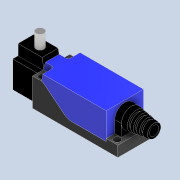
# Autodesk Inventor part: High Voltage Limit Switch
Saved by Autodesk Inventor 2022 (Build 260153000, 153)
## iProperties
Created: 2021-10-24
Part Number: High Voltage Limit Switch
Material: Generic
Document SubType Name: Modeling
Designer: Coy
Density: 1 g/cm^3
Appearance: Anodized - Black
Author: Coy
Autodesk Inventor part; units mm, degrees
ref_plane "YZ Plane" through (0, 0, 0) normal (1, 0, 0) x (0, 1, 0)
sketch "Sketch1" plane through (0, 0, 0) normal (0, 1, 0) x (-1, 0, 0)
  line L0 (0, 0) -> (64, 0)
  line L1 (64, 0) -> (64, 28)
  line L2 (64, 28) -> (0, 28)
  line L3 (0, 28) -> (0, 0)
  dimension "d0" = 64
  dimension "d1" = 28
  constraints: 8 end point, 2 parallel, 1 horizontal, 1 perpendicular
  measures "d0" distance of L1.end L2.end
  measures "d1" distance of L2.end L0.start
extrude "Extrusion1" add sketch "Sketch1" along normal blind 21
sketch "Sketch2" plane through (0, 0, 0) normal (0, 0, -1) x (-1, 0, 0)
  line L0 (0, 0) -> (64, 0) projected
  line L1 (64, 0) -> (64, 21) projected
  line L2 (0, 21) -> (64, 21) projected
  line L3 (0, 0) -> (0, 21) projected
  line L4 (0, 0) -> (0, 21) projected
  line L5 (0, 8) -> (8.75, 8)
  line L6 (0, 0) -> (0, 21) projected
  line L7 (8.75, 6) -> (34.2422, 6)
  line L8 (8.75, 6) -> (8.75, 8)
  line L9 (64, 21) -> (57.2016, 21)
  line L10 (64, 21) -> (0, 21) projected
  line L11 (55.9522, 20.5617) -> (40.4891, 8.1913)
  arc A0 (34.2422, 6) -> (40.4891, 8.1913) centre (34.2422, 16) ccw
  arc A1 (57.2016, 21) -> (55.9522, 20.5617) centre (57.2016, 19) ccw
  point P0 (37.75, 6)
  point P1 (56.5, 21)
  point P2 (57.2016, 21)
  dimension "d4" = 8.75
  dimension "d5" = 8
  dimension "d6" = 29
  dimension "d7" = 2
  dimension "d8" = 7.5
  dimension "d9" = 10
  dimension "d10" = 2
  constraints: 10 end point, 6 point on line, 4 point on circle, 4 tangent, 3 perpendicular, 2 centre point, 1 horizontal
  measures "d4" distance of L5.start L5.end
  measures "d5" distance between parallel lines of L0 L5
  measures "d6" distance of L7.start point (37.75, 6)
  measures "d7" distance of L7.start L5.end
  measures "d8" distance of L1.end point (56.5, 21)
  measures "d9" radius of A0
  measures "d10" radius of A1
extrude "Extrusion2" cut sketch "Sketch2" against normal up to next contours L3 L2 A1 L11 A0 L7 L8 L5
ref_plane "Work Plane1" through (0, 26, 0) normal (0, -1, 0) x (1, 0, 0)
sketch "Sketch3" plane through (0, 26, 0) normal (0, -1, 0) x (1, 0, 0)
  line L0 (-64, 28) -> (0, 28) projected
  line L1 (-8.75, 28) -> (-8.75, 0)
  line L2 (0, 0) -> (0, 28) projected
  line L3 (-57.2016, 28) -> (-57.2016, 0) projected
  line L4 (-57.2016, 0) -> (-55.9522, 0) projected
  line L5 (-55.9522, 0) -> (-40.4891, 0) projected
  line L6 (-34.2422, 0) -> (-40.4891, 0) projected
  line L7 (-34.2422, 0) -> (-8.75, 0) projected
  line L8 (-64, 0) -> (-64, 28) projected
  line L9 (-64, 20) -> (-57.1916, 20)
  line L10 (-57.2016, 20) -> (-57.2016, 8)
  line L11 (-57.1916, 8) -> (-64, 8)
  line L12 (-64, 8) -> (-64, 20)
  line L13 (-0.01, 0) -> (-0.01, 27.99)
  line L14 (-0.01, 27.99) -> (-63.99, 27.99)
  line L15 (-63.99, 27.99) -> (-63.99, 0)
  line L16 (-7.5, 0.01) -> (-34.0284, 0.01)
  line L17 (-34.0284, 0.01) -> (-40.2248, 0.01)
  line L18 (-40.2248, 0.01) -> (-55.955, 0.01)
  line L19 (-55.955, 0.01) -> (-57.1916, 0.01)
  line L20 (-57.1916, 0.01) -> (-57.1916, 28)
  point P0 (-8.75, 27.99)
  point P1 (-57.2016, 27.99)
  point P2 (-63.99, 20)
  point P3 (-63.99, 8)
  point P4 (-8.75, 0.01)
  point P5 (-57.1916, 27.99)
  dimension "d14" = 8.75
  dimension "d15" = 12
  dimension "d16" = 8
  dimension "d17" = 0.01
  dimension "d18" = 0.01
  constraints: 26 end point, 7 point on line, 2 parallel, 1 horizontal, 1 perpendicular, 1 vertical, 6 other
  measures "d14" distance between parallel lines of L2 L1
  measures "d15" distance between parallel lines of L11 L9
  measures "d16" distance between parallel lines of L0 L9
  measures "d17" distance between parallel lines of L0 L14
  measures "d18" distance between parallel lines of L5 L18
extrude "Extrusion3" add sketch "Sketch3" along normal up to next contours L9 L3 L11 L15 | L14 L1 L16 L17 L18 L19 L20 | L9 L20 L11 L3
sketch "Sketch4" plane through (-64, 0, 0) normal (-1, 0, 0) x (0, 0, 1)
  line L0 (3.8444, 20.5) -> (23.8444, 20.5)
  line L1 (23.8444, 20.5) -> (23.8444, 0.5)
  line L2 (23.8444, 0.5) -> (3.8444, 0.5)
  line L3 (3.8444, 0.5) -> (3.8444, 20.5)
  line L4 (3.8444, 20.5) -> (-0.3111, 20.5) construction
  line L5 (3.8444, 20.5) -> (3.8444, 21) construction
  line L6 (0, 21) -> (28, 21) construction
  line L7 (23.8444, 0.5) -> (23.8444, 0) construction
  line L8 (28, 0) -> (0, 0) construction
  line L9 (23.8444, 0.5) -> (28, 0.5) construction
  line L10 (28, 0) -> (28, 8) construction
  dimension "d21" = 20
  dimension "d22" = 20
  constraints: 16 end point, 5 parallel, 3 point on line, 2 horizontal, 2 perpendicular, 1 vertical
  measures "d21" distance of L1.end L2.end
  measures "d22" distance of L0.end L1.end
extrude "Extrusion4" add sketch "Sketch4" along normal blind 19
sketch "Sketch5" plane through (-64, 20.5, 23.8444) normal (0, 1, 0) x (1, 0, 0)
  line L0 (-19, 20) -> (-19, 0) projected
  line L1 (0, 23.8444) -> (0, -4.1556) projected
  line L2 (-19, 15.9795) -> (0, 15.9795)
  line L3 (0, 15.9795) -> (0, 3.9795)
  line L4 (0, 3.9795) -> (-19, 3.9795)
  line L5 (-19, 3.9795) -> (-19, 15.9795)
  line L6 (-9.5, 15.9795) -> (-9.5, 20) construction
  line L7 (0, 20) -> (-19, 20) construction
  line L8 (-9.5, 3.9795) -> (-9.5, -0.041) construction
  point P0 (64, 23.8444)
  point P1 (-19, 3.9795)
  point P2 (0, 15.9795)
  dimension "d25" = 12
  constraints: 12 end point, 3 midpoint, 3 point on line, 2 parallel, 1 collinear, 1 horizontal, 1 perpendicular
  measures "d25" distance of L2.end L3.end
chamfer "Chamfer1" distance 5 angle 10 1 edges at (-63.99, 26, 14) measured on face at (-63.99, 25.5, 14)
chamfer "Chamfer2" distance 5 angle 10 1 edges at (-57.1916, 26, 23.995) measured on face at (-57.1916, 25.5, 23.995)
chamfer "Chamfer3" distance 5 angle 10 1 edges at (-57.1916, 26, 4.005) measured on face at (-57.1916, 25.5, 4.005)
chamfer "Chamfer4" distance 5 angle 10 2 edges at (-56.7507, 26, 20) (-60.15, 26, 20) measured on face at (-60.15, 25.5, 20) measured on face at (-56.7507, 25.5, 20)
chamfer "Chamfer5" distance 5 angle 10 2 edges at (-60.15, 26, 8) (-56.7507, 26, 8) measured on face at (-60.15, 25.5, 8) measured on face at (-56.7507, 25.5, 8)
extrude "Extrusion5" add sketch "Sketch5" along normal blind 8
chamfer "Chamfer6" distance 5 angle 10 1 edges at (-64, 28.5, 13.8649) measured on face at (-64, 28, 13.8649)
fillet "Fillet1" radius 2 5 edges at (-57.1916, 21, 8) (-56.7507, 23.5001, 8.4408) (-57.1916, 21.0001, 20) (-57.1916, 21, 20) (-56.7507, 23.5001, 19.5592)
sketch "Sketch6" plane through (0, 0, 0) normal (0, -1, 0) x (1, 0, 0)
  line L0 (-64, 0) -> (-64, 28) projected
  line L1 (0, 0) -> (-64, 0) projected
  line L2 (0, 28) -> (0, 0) projected
  line L3 (-64, 28) -> (0, 28) projected
  line L4 (-60, 3.5) -> (-4, 3.5) construction
  line L5 (-4, 3.5) -> (-4, 24.5) construction
  line L6 (-4, 24.5) -> (-60, 24.5) construction
  line L7 (-60, 24.5) -> (-60, 3.5) construction
  line L8 (-60, 3.5) -> (-64, 3.5) construction
  line L9 (-64, 0) -> (-64, 7.8649) construction
  line L10 (-60, 3.5) -> (-60, 0) construction
  line L11 (-4, 24.5) -> (0, 24.5) construction
  line L12 (0, 0) -> (0, 28) construction
  line L13 (-4, 24.5) -> (-4, 28) construction
  circle A0 centre (-4, 24.5) radius 2.5
  circle A1 centre (-4, 3.5) radius 2.5
  circle A2 centre (-60, 24.5) radius 2.5
  circle A3 centre (-60, 3.5) radius 2.5
  dimension "d47" = 56
  dimension "d48" = 21
  dimension "d49" = 5
  dimension "d50" = 5
  dimension "d51" = 5
  dimension "d52" = 5
  constraints: 16 end point, 5 perpendicular, 4 centre point, 4 coincident, 4 parallel, 4 point on line, 1 horizontal
  measures "d47" distance of L6.end L5.end
  measures "d48" distance of L5.end L4.end
  measures "d49" diameter of A0
  measures "d50" diameter of A2
  measures "d51" diameter of A3
  measures "d52" diameter of A1
extrude "Extrusion6" cut sketch "Sketch6" against normal up to next contours A0 | A1 | A2 | A3
thread "Thread1" size "M5x0.8" class "6H" standard "ANSI Metric M Profile" full length
thread "Thread2" size "M5x0.8" class "6H" standard "ANSI Metric M Profile" full length
thread "Thread3" size "M5x0.8" class "6H" standard "ANSI Metric M Profile" full length
thread "Thread4" size "M5x0.8" class "6H" standard "ANSI Metric M Profile" full length
sketch "Sketch7" plane through (-8.75, 26, 27.99) normal (1, 0, 0) x (0, 0, -1)
  line L0 (27.99, -18) -> (-0.01, -18) projected
  line L1 (13.99, -18) -> (13.99, 0) construction
  line L2 (27.98, 0) -> (0, 0) construction
  circle A0 centre (13.99, -9) radius 7.5
  line L3 (21.49, -9) -> (21.49, -18)
  line L4 (6.49, -9) -> (6.49, -18)
  point P0 (27.99, -26)
  dimension "d63" = 15
  constraints: 6 end point, 3 midpoint, 2 perpendicular, 2 point on circle, 2 point on line, 1 centre point
  measures "d63" diameter of A0
extrude "Extrusion7" add sketch "Sketch7" along normal blind 5
ref_plane "Work Plane2" through (-64, 0, 14) normal (0, 0, 1) x (1, 0, 0)
sketch "Sketch8" plane through (-64, 0, 14) normal (0, 0, 1) x (1, 0, 0)
  line L0 (55.25, 17) -> (60.25, 17) construction
  line L1 (60.25, 17) -> (97.4201, 17)
  line L2 (77.25, 17) -> (77.25, 22)
  line L3 (60.25, 17) -> (60.25, 24.5) projected
  line L4 (74.0613, 20.9528) -> (74.0613, 22.4689)
  line L5 (72.0613, 21.2469) -> (72.0613, 22.763)
  line L6 (70.0613, 21.541) -> (70.0613, 23.0572)
  line L7 (68.0613, 21.8351) -> (68.0613, 23.3513)
  line L8 (66.0613, 22.1293) -> (66.0613, 23.6454)
  line L9 (64.0613, 22.4234) -> (64.0613, 23.9395)
  line L10 (64.0613, 23.9395) -> (60.25, 24.5)
  line L11 (68.0613, 23.3513) -> (66.0613, 23.6454)
  line L12 (77.25, 22) -> (74.0613, 22.4689)
  line L13 (72.0613, 22.763) -> (70.0613, 23.0572)
  line L14 (72.0613, 21.2469) -> (74.0613, 20.9528)
  line L15 (64.0613, 22.4234) -> (66.0613, 22.1293)
  line L16 (68.0613, 21.8351) -> (70.0613, 21.541)
  point P0 (64, 0)
  dimension "d67" = 5
  dimension "d68" = 17
  dimension "d69" = 2
  dimension "d70" = 2
  dimension "d71" = 2
  dimension "d72" = 2
  dimension "d73" = 2
  constraints: 30 end point, 5 parallel, 1 horizontal, 1 perpendicular, 1 point on line, 1 vertical
  measures "d67" distance of L2.start L2.end
  measures "d68" distance between parallel lines of L3 L2
  measures "d69" distance between parallel lines of L4 L5
  measures "d70" distance between parallel lines of L5 L6
  measures "d71" distance between parallel lines of L6 L7
  measures "d72" distance between parallel lines of L7 L8
  measures "d73" distance between parallel lines of L8 L9
revolve "Revolution1" add sketch "Sketch8" angle 360 about axis through (-3.75, 17, 14) along (1, 0, 0)
sketch "Sketch9" plane through (13.25, 17, 14) normal (1, 0, 0) x (0, 0, -1)
  circle A0 centre (0, 0) radius 3.5
  point P0 (14, -17)
  dimension "d76" = 7
  constraints: 1 centre point
  measures "d76" diameter of A0
extrude "Extrusion8" cut sketch "Sketch9" against normal blind 20
sketch "Sketch10" plane through (-64, 28.5, 23.8444) normal (0, 1, 0) x (1, 0, 0)
  line L0 (-19, 20) -> (-19, 0) construction
  line L1 (-19, 10) -> (-0.8816, 9.9795) construction
  line L2 (-0.8816, 15.9795) -> (-0.8816, 3.9795) construction
  circle A0 centre (-8.5, 9.9881) radius 3
  circle A1 centre (4, 20.3444) radius 2.5 projected
  point P0 (64, 23.8444)
  dimension "d79" = 6
  dimension "d80" = 12.5
  constraints: 2 end point, 2 midpoint, 1 centre point, 1 point on line
  measures "d79" diameter of A0
  measures "d80" horizontal distance of A1.centre A0.centre
extrude "Extrusion9" add sketch "Sketch10" along normal blind 10.35 contours A0
equation "\"d50\" = d49"
equation "\"d51\" = d49"
equation "\"d52\" = d49"
body "Solid1"
